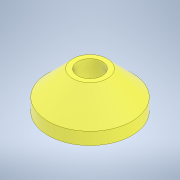
# Autodesk Inventor part: Apoio da Morsa
Saved by Autodesk Inventor 2021 (Build 250183000, 183)
## iProperties
Created: 2021-05-13
Part Number: Apoio da Morsa
Material: Genérico
Document SubType Name: Modeling
Designer: rubia
Density: 1 g/cm^3
Appearance: Suave - Amarelo
Author: rubia
Autodesk Inventor part; units mm, degrees
ref_plane "YZ Plane" through (0, 0, 0) normal (1, 0, 0) x (0, 1, 0)
ref_plane "XZ Plane" through (0, 0, 0) normal (0, 1, 0) x (-1, 0, 0)
ref_plane "XY Plane" through (0, 0, 0) normal (0, 0, 1) x (1, 0, 0)
sketch "Esboço1" plane through (0, 0, 0) normal (0, 0, 1) x (1, 0, 0)
  line L0 (0, 0) -> (-34, 0)
  line L1 (-34, 0) -> (-34, 10)
  line L2 (0, 0) -> (0, 15)
  line L3 (0, 15) -> (-10, 15)
  line L4 (-10, 15) -> (-10, 30)
  line L5 (-34, 10) -> (-14, 30)
  line L6 (-10, 30) -> (-14, 30)
  dimension "d0" = 34
  dimension "d1" = 10
  dimension "d2" = 15
  dimension "d3" = 10
  dimension "d4" = 15
  dimension "d5" = 45
  constraints: 14 end point, 3 perpendicular, 2 horizontal, 1 vertical
  measures "d0" distance of L0.start L0.end
  measures "d1" distance of L0.end L1.end
  measures "d2" distance of L0.start L2.end
  measures "d3" distance of L2.end L3.end
  measures "d4" distance of L3.end L4.end
  measures "d5" angle of L0 L5
revolve "Revolução1" add sketch "Esboço1" angle 360 about axis through (0, 0, 0) along (0, 1, 0)
